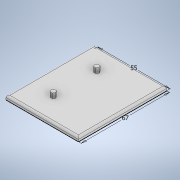
# Autodesk Inventor part: Star_Wars_Base
Saved by Autodesk Inventor 2020.3 (Build 243373000, 373)
## iProperties
Created: 2021-03-09
Part Number: Star_Wars_Base
Material: Generic
Document SubType Name: Modeling
Designer: super
Density: 1 g/cm^3
Appearance: Default
Author: super
Autodesk Inventor part; units mm, degrees
ref_plane "YZ Plane" through (0, 0, 0) normal (1, 0, 0) x (0, 1, 0)
ref_plane "XZ Plane" through (0, 0, 0) normal (0, 1, 0) x (-1, 0, 0)
ref_plane "XY Plane" through (0, 0, 0) normal (0, 0, 1) x (1, 0, 0)
sketch "Sketch1" plane through (0, 0, 0) normal (0, 1, 0) x (-1, 0, 0)
  line L0 (0, 0) -> (-55, 0)
  line L1 (-55, 0) -> (-55, -67)
  line L2 (-55, -67) -> (0, -67)
  line L3 (0, -67) -> (0, 0)
  dimension "d0" = 55
  dimension "d1" = 67
  constraints: 8 end point, 2 parallel, 1 horizontal, 1 perpendicular
  measures "d0" distance of L2.end L1.end
  measures "d1" distance of L1.end L0.end
extrude "Extrusion1" add sketch "Sketch1" along normal blind 3
sketch "Sketch2" plane through (0, 3, 0) normal (0, 1, 0) x (1, 0, 0)
  line L0 (55, 0) -> (55, 67) projected
  line L1 (0, 0) -> (55, 0) projected
  line L2 (20.8, 17) -> (19.9, 15.4412)
  line L3 (19.9, 15.4412) -> (18.1, 15.4412)
  line L4 (18.1, 15.4412) -> (17.2, 17)
  line L5 (17.2, 17) -> (18.1, 18.5588)
  line L6 (18.1, 18.5588) -> (19.9, 18.5588)
  line L7 (19.9, 18.5588) -> (20.8, 17)
  line L8 (20.8, 50) -> (19.9, 48.4412)
  line L9 (19.9, 48.4412) -> (18.1, 48.4412)
  line L10 (18.1, 48.4412) -> (17.2, 50)
  line L11 (17.2, 50) -> (18.1, 51.5588)
  line L12 (18.1, 51.5588) -> (19.9, 51.5588)
  line L13 (19.9, 51.5588) -> (20.8, 50)
  point P0 (19, 17)
  point P1 (19, 50)
  constraints: 24 end point, 26 other
extrude "Extrusion2" add sketch "Sketch2" along normal blind 3.7
fillet "Fillet1" radius 1.5 4 edges at (0, 3, -33.5) (27.5, 3, 0) (55, 3, -33.5) (27.5, 3, -67)
body "Solid1"
